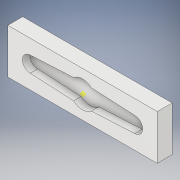
# Autodesk Inventor part: micro_horn_test
Saved by Autodesk Inventor 2018 (Build 220112000, 112)
## iProperties
Created: 2015-02-12
Part Number: micro_horn_test
Material: Generic
Document SubType Name: Modeling
Designer: scwu
Density: 1 g/cm^3
Appearance: Default
Sending System: SolidWorks 2013
Last Author: Димтрий
Last Saved: 2015-02-27
Author: scwu
Autodesk Inventor part; units mm, degrees
ref_plane "YZ Plane" through (0, 0, 0) normal (1, 0, 0) x (0, 1, 0)
ref_plane "XZ Plane" through (0, 0, 0) normal (0, 1, 0) x (-1, 0, 0)
ref_plane "XY Plane" through (0, 0, 0) normal (0, 0, 1) x (1, 0, 0)
sketch "Sketch2" plane through (0, 0, 0) normal (0, 0, 1) x (1, 0, 0)
  line L0 (-20, 6) -> (20, 6)
  line L1 (20, 6) -> (20, -6)
  line L2 (20, -6) -> (-20, -6)
  line L3 (-20, -6) -> (-20, 6)
  line L4 (-20, 6) -> (20, -6) construction
  line L5 (20, 6) -> (-20, -6) construction
  point P0 (0, 0)
  dimension "d0" = 40
  dimension "d1" = 12
  constraints: 12 end point, 2 midpoint, 2 parallel, 1 horizontal, 1 perpendicular
  measures "d0" distance of L1.end L2.end
  measures "d1" distance of L0.end L1.end
extrude "Extrusion1" add sketch "Sketch2" against normal blind 4
sketch "Sketch3" plane through (0, 0, 0) normal (0, 0, 1) x (1, 0, 0)
  line L0 (0, 0) -> (16.1, 0) construction
  line L1 (0, 0) -> (16.1, 0) construction
  arc A0 (14, -2.1) -> (14, 2.1) centre (14, 0) ccw
  line L2 (2.3812, 0) -> (2.3812, 2.7) construction
  line L3 (2.3812, 2.7) -> (14, 2.1)
  line L4 (2.3812, -2.7) -> (14, -2.1)
  line L5 (0, 0) -> (0, 3.6) construction
  arc A1 (-14, 2.1) -> (-14, -2.1) centre (-14, 0) ccw
  line L6 (-2.3812, 2.7) -> (-14, 2.1)
  line L7 (-2.3812, -2.7) -> (-14, -2.1)
  arc A2 (2.3812, 2.7) -> (-2.3812, 2.7) centre (0, 0) ccw
  arc A3 (-2.3812, -2.7) -> (2.3812, -2.7) centre (0, 0) ccw
  dimension "d10" = 16.1
  dimension "d12" = 2.7
  constraints: 16 end point, 10 point on circle, 7 symmetric about line, 4 centre point, 2 coincident, 2 horizontal, 2 point on line, 1 collinear, 1 perpendicular, 1 vertical, 1 other
  measures "d10" distance of L0.start L0.end
  measures "d12" distance of L2.end L2.start
extrude "Extrusion3" cut sketch "Sketch3" against normal blind 2
body "Solid1"
